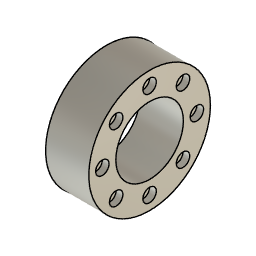
Link7 v8 (Autodesk Fusion 360 design; units mm, degrees)
Autodesk Fusion 360 part; units mm, degrees
note: some values were not read from the file. Set by a fixed rule: which sketch regions a step uses.
sketch "Boceto1" plane through (0, 0, 0) normal (0, 0, 1) x (1, 0, 0)
  circle A0 centre (0, 0) radius 45
  dimension "d1" = 90
  constraint coincident A0.centre origin
  measures "d1" diameter of A0
extrude "Extruir1" add sketch "Boceto1" along normal blind 32
sketch "Boceto2" plane through (0, 0, 32) normal (0, 0, 1) x (1, 0, 0)
  circle A0 centre (0, 0) radius 45
  circle A1 centre (0, 0) radius 25
  dimension "d4" = 50
  constraint coincident A0.centre A1.centre
  measures "d4" diameter of A1
extrude "Extruir2" cut sketch "Boceto2" against normal blind 60 contours A1
sketch "Boceto3" plane through (0, 0, 0) normal (0, 0, -1) x (-1, 0, 0)
  circle A0 centre (0, 0) radius 25
  circle A1 centre (0, 0) radius 45
  circle A2 centre (0, 0) radius 35
  line L0 (0, 0) -> (24.7487, 24.7487)
  line L1 (0, 0) -> (35, 0) construction
  line L2 (0, 0) -> (-24.7487, 24.7487)
  line L3 (0, 0) -> (-24.7487, -24.7487)
  line L4 (0, 0) -> (24.7487, -24.7487)
  circle A3 centre (-24.7487, 24.7487) radius 5
  circle A4 centre (0, 35) radius 5
  circle A5 centre (24.7487, 24.7487) radius 5
  circle A6 centre (-35, 0) radius 5
  circle A7 centre (35, 0) radius 5
  circle A8 centre (24.7487, -24.7487) radius 5
  circle A9 centre (-24.7487, -24.7487) radius 5
  circle A10 centre (0, -35) radius 5
  point P0 (-24.7487, 24.7487)
  dimension "d7" = 70
  dimension "d8" = 45
  dimension "d9" = 35
  dimension "d10" = 35
  dimension "d11" = 10
  dimension "d12" = 10
  dimension "d13" = 10
  dimension "d14" = 10
  dimension "d15" = 10
  dimension "d16" = 10
  dimension "d17" = 10
  dimension "d18" = 10
  constraint coincident A0.centre A1.centre
  constraint horizontal L1
  constraint perpendicular L0 L2
  constraint coincident A2 L3.end
  constraint perpendicular L2 L3
  constraint coincident A2 L4.end
  constraint perpendicular L3 L4
  constraint coincident P0 L2.end
  constraint coincident A2 A4.centre
  constraint coincident L0.end A5.centre
  constraint coincident A2 A6.centre
  constraint coincident L1.end A7.centre
  constraint coincident L4.end A8.centre
  constraint coincident L3.end A9.centre
  constraint coincident A2 A10.centre
  measures "d7" diameter of A2
  measures "d8" angle of L0 L1
  measures "d9" distance of A0.centre L0.end
  measures "d10" distance of A0.centre P0
  measures "d11" diameter of A3
  measures "d12" diameter of A4
  measures "d13" diameter of A5
  measures "d14" diameter of A6
  measures "d15" diameter of A7
  measures "d16" diameter of A8
  measures "d17" diameter of A9
  measures "d18" diameter of A10
extrude "Extruir3" cut sketch "Boceto3" against normal blind 5 contours A2 L0 A5 | A2 L0 A5 | A2 L4 A8 | A2 L4 A8 | A2 L2 A3 | A2 L2 A3 | A2 A5 | A2 L3 A9 | A2 L3 A9 | A2 A8 | A2 A3 | A2 A4 | A2 A4 | A2 A7 | A2 A7 | A2 A9 | A2 A10 | A2 A10 | A2 A6 | A2 A6
move_body "Desplazar1" bodies 1 to x (1, 0, 0) y (0, 0, 1) z (0, -1, 0) at (0, -45, 45)
move_body "Desplazar2" bodies 1 to x (1, 0, 0) y (0, 1, 0) z (0, 0, 1) at (-0.0001, 0, -45.0001)
move_body "Desplazar3" bodies 1 to x (1, 0, 0) y (0, 1, 0) z (0, 0, 1) at (0, 45, 0)
sketch "Sketch4" plane through (0, 0, 0) normal (1, 0, 0) x (0, 1, 0)
  line L0 (-32, 0) -> (0, 0)
  constraint coincident L0.end origin
  constraint horizontal L0
move_body "Move4" bodies 1 to x (1, 0, 0) y (0, 1, 0) z (0, 0, 1) at (0, 32, 0)
sketch "Sketch5" plane through (0, 0, 0) normal (0, 0, 1) x (1, 0, 0)
  line L0 (-45.0001, 32) -> (44.9999, 32)
  dimension "d21" = 32
  measures "d21" distance of L0 origin
